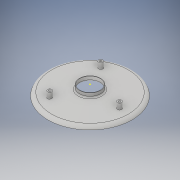
# Autodesk Inventor part: Alojamento do Sensor de Temperatura e Umidade - tampa
Saved by Autodesk Inventor 2019.4 (Build 234330000, 330)
## iProperties
Created: 2021-02-17
Part Number: Alojamento do Sensor de Temperatura e Umidade - tampa
Material: Genérico
Document SubType Name: Modeling
Designer: Lattes
Density: 1 g/cm^3
Appearance: Padrão
Author: Lattes
Autodesk Inventor part; units mm, degrees
ref_plane "YZ Plane" through (0, 0, 0) normal (1, 0, 0) x (0, 1, 0)
ref_plane "XZ Plane" through (0, 0, 0) normal (0, 1, 0) x (-1, 0, 0)
ref_plane "XY Plane" through (0, 0, 0) normal (0, 0, 1) x (1, 0, 0)
sketch "Esboço1" plane through (0, 0, 0) normal (0, 0, 1) x (1, 0, 0)
  line L0 (15, 13) -> (15, 9.8301)
  line L1 (16.8229, 7.838) -> (54.5312, 4.4861)
  line L2 (14.4, 12.4) -> (14.4, 9.2811)
  line L3 (16.2229, 7.2889) -> (53.9312, 3.9371)
  line L4 (0, 0) -> (0, 5.451)
  arc A0 (59.0428, 0) -> (53.9312, 3.9371) centre (53.4, -2.0394) ccw
  arc A1 (59.812, 0) -> (54.5312, 4.4861) centre (54, -1.4903) ccw
  line L5 (59.812, 0) -> (59.0428, 0)
  arc A2 (15, 9.8301) -> (16.8229, 7.838) centre (17, 9.8301) ccw
  arc A3 (14.4, 9.2811) -> (16.2229, 7.2889) centre (16.4, 9.2811) ccw
  line L6 (14.4, 12.4) -> (14.4, 13.9165)
  line L7 (15, 12.4) -> (15, 13.9165)
  line L8 (15, 13.9165) -> (14.4, 13.9165)
  point P0 (60, 4)
  point P1 (15, 14)
  point P2 (15, 8)
  dimension "d5" = 6
  dimension "d7" = 6
  dimension "d8" = 2
  constraints: 18 end point, 8 point on circle, 6 tangent, 5 point on line, 4 centre point, 2 equal radius, 2 vertical, 1 horizontal, 1 perpendicular, 1 other
  measures "d5" distance of point (15, 14) point (15, 8)
  measures "d7" radius of A0
  measures "d8" radius of A2
revolve "Revolução1" add sketch "Esboço1" angle 360 about axis through (0, 0, 0) along (0, 1, 0)
sketch "Esboço3" plane through (0, 13.9165, 0) normal (0, 1, 0) x (1, 0, 0)
  line L0 (0, 0) -> (42, 0)
  circle A0 centre (42, 0) radius 1.5
  circle A1 centre (42, 0) radius 3
  dimension "d18" = 42
  dimension "d19" = 3
  dimension "d25" = 6
  constraints: 2 centre point, 2 coincident, 2 end point, 1 horizontal
  measures "d18" distance of L0.start L0.end
  measures "d19" diameter of A0
  measures "d25" diameter of A1
sketch "Esboço4" plane through (0, 13.9165, 0) normal (0, 1, 0) x (1, 0, 0)
  point P0 (0, 0)
extrude "Extrusão3" add sketch "Esboço3" against normal blind 10
pattern_circular "Padrão circular3" count 3 over 360 about axis through (0, 6.162, 0) along (0, -1, 0) of "Extrusão3"
